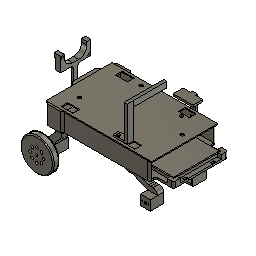
NatBot_V1 (Autodesk Fusion 360 design; units mm, degrees)
Autodesk Fusion 360 part; units mm, degrees
note: some values were not read from the file. Set by a fixed rule: which face or edge a step refers to.
(part 1 of 5)
sketch "MiniBot_v1" plane through (0, 0, 0) normal (0, 1, 0) x (1, 0, 0)
  line L0 (130.81, 3.81) -> (114.3, 3.81)
  circle A0 centre (147.6502, 58.6486) radius 2.54
  line L1 (114.3, 3.81) -> (114.3, 13.97)
  line L2 (130.81, 13.97) -> (130.81, 3.81)
  line L3 (114.3, 13.97) -> (130.81, 13.97)
  circle A1 centre (21.2344, 29.4894) radius 2.54
  line L4 (0, 0) -> (160, 0)
  line L5 (114.3, 86.36) -> (114.3, 96.52)
  line L6 (19.05, 96.52) -> (36.83, 96.52)
  line L7 (160, 0) -> (160, 100)
  line L8 (114.3, 96.52) -> (130.81, 96.52)
  line L9 (36.83, 96.52) -> (36.83, 86.36)
  circle A2 centre (102.5398, 7.1374) radius 2.54
  line L10 (36.83, 13.97) -> (36.83, 3.81)
  line L11 (19.05, 13.97) -> (36.83, 13.97)
  line L12 (19.05, 86.36) -> (19.05, 96.52)
  line L13 (36.83, 3.81) -> (19.05, 3.81)
  line L14 (130.81, 86.36) -> (114.3, 86.36)
  line L15 (19.05, 3.81) -> (19.05, 13.97)
  line L16 (130.81, 96.52) -> (130.81, 86.36)
  circle A3 centre (122.9106, 82.4992) radius 2.54
  line L17 (160, 100) -> (0, 100)
  line L18 (36.83, 86.36) -> (19.05, 86.36)
  circle A4 centre (52.2224, 92.0496) radius 2.54
  line L19 (0, 100) -> (0, 0)
extrude "Extrude1" add sketch "MiniBot_v1" along normal blind 1.57 makes body 1
sketch "Sketch1" plane through (0, 0, 0) normal (0, -1, 0) x (1, 0, 0) in component "battery"
  line L0 (19.05, -3.81) -> (36.83, -3.81)
  line L1 (36.83, -3.81) -> (36.83, -13.97)
  line L2 (36.83, -13.97) -> (19.05, -13.97)
  line L3 (19.05, -13.97) -> (19.05, -3.81)
  circle A0 centre (122.9106, -82.4992) radius 2.54
  circle A1 centre (52.2224, -92.0496) radius 2.54
  line L4 (130.81, -96.52) -> (114.3, -96.52)
  line L5 (114.3, -96.52) -> (114.3, -86.36)
  line L6 (114.3, -86.36) -> (130.81, -86.36)
  line L7 (130.81, -86.36) -> (130.81, -96.52)
  line L8 (36.83, -86.36) -> (36.83, -96.52)
  line L9 (36.83, -96.52) -> (19.05, -96.52)
  line L10 (19.05, -96.52) -> (19.05, -86.36)
  line L11 (19.05, -86.36) -> (36.83, -86.36)
  circle A2 centre (102.5398, -7.1374) radius 2.54
  circle A3 centre (21.2344, -29.4894) radius 2.54
  circle A4 centre (147.6502, -58.6486) radius 2.54
  line L12 (114.3, -13.97) -> (114.3, -3.81)
  line L13 (114.3, -3.81) -> (130.81, -3.81)
  line L14 (130.81, -3.81) -> (130.81, -13.97)
  line L15 (130.81, -13.97) -> (114.3, -13.97)
  line L16 (0, 0) -> (0, -100)
  line L17 (0, -100) -> (160, -100)
  line L18 (160, -100) -> (160, 0)
  line L19 (160, 0) -> (0, 0)
  line L20 (174, 0) -> (224.77, 0)
  line L21 (224.77, 0) -> (224.77, -71)
  line L22 (224.77, -71) -> (174, -71)
  line L23 (174, -71) -> (174, 0)
  dimension "d3" = 50.77
  dimension "d4" = 71
  constraint horizontal L20
  constraint vertical L21
  constraint horizontal L22
  constraint vertical L23
  measures "d3" distance of L20.start L20.end
  measures "d4" distance of L20.end L21.end
extrude "Extrude1'" add sketch "Sketch1" along normal blind 6 separate body contours L20 L21 L22 L23 makes body 2 in component "battery"
sketch "Sketch1 (2)" plane through (0, 0, 0) normal (0, -1, 0) x (1, 0, 0) in component "Arduino"
  line L0 (19.05, -3.81) -> (36.83, -3.81)
  line L1 (36.83, -3.81) -> (36.83, -13.97)
  line L2 (36.83, -13.97) -> (19.05, -13.97)
  line L3 (19.05, -13.97) -> (19.05, -3.81)
  circle A0 centre (122.9106, -82.4992) radius 2.54
  circle A1 centre (52.2224, -92.0496) radius 2.54
  line L4 (130.81, -96.52) -> (114.3, -96.52)
  line L5 (114.3, -96.52) -> (114.3, -86.36)
  line L6 (114.3, -86.36) -> (130.81, -86.36)
  line L7 (130.81, -86.36) -> (130.81, -96.52)
  line L8 (36.83, -86.36) -> (36.83, -96.52)
  line L9 (36.83, -96.52) -> (19.05, -96.52)
  line L10 (19.05, -96.52) -> (19.05, -86.36)
  line L11 (19.05, -86.36) -> (36.83, -86.36)
  circle A2 centre (102.5398, -7.1374) radius 2.54
  circle A3 centre (21.2344, -29.4894) radius 2.54
  circle A4 centre (147.6502, -58.6486) radius 2.54
  line L12 (114.3, -13.97) -> (114.3, -3.81)
  line L13 (114.3, -3.81) -> (130.81, -3.81)
  line L14 (130.81, -3.81) -> (130.81, -13.97)
  line L15 (130.81, -13.97) -> (114.3, -13.97)
  line L16 (0, 0) -> (0, -100)
  line L17 (0, -100) -> (160, -100)
  line L18 (160, -100) -> (160, 0)
  line L19 (160, 0) -> (0, 0)
  line L20 (92.1, -65.68) -> (38.1, -65.68)
  line L21 (38.1, -65.68) -> (38.1, -27.68)
  line L22 (38.1, -27.68) -> (92.1, -27.68)
  line L23 (92.1, -27.68) -> (92.1, -65.68)
  line L24 (92.1, -65.68) -> (38.1, -27.68) construction
  line L25 (38.1, -65.68) -> (92.1, -27.68) construction
  point P0 (65.1, -46.68)
  dimension "d7" = 54
  dimension "d8" = 38
  dimension "d9" = 27.68
  dimension "d10" = 38.1
  constraint horizontal L20
  constraint perpendicular L20 L21
  constraint parallel L20 L22
  constraint parallel L21 L23
  constraint coincident L24 P0
  constraint coincident L25 P0
  measures "d7" distance of L21.end L22.end
  measures "d8" distance of L20.end L21.end
  measures "d9" distance of L19 L22
  measures "d10" distance of L16 L21
extrude "Extrude1''" add sketch "Sketch1 (2)" along normal blind 11.3 separate body contours L20 L21 L22 L23 makes body 3 in component "Arduino"
fillet "Fillet1" radius 1 12 edges at (224.77, 0, -35.5) (224.77, -6, -35.5) (224.77, -3, 0) (199.385, 0, 0) (199.385, -6, 0) (199.385, 0, -71) (224.77, -3, -71) (199.385, -6, -71) (174, -3, -71) (174, -6, -35.5) (174, 0, -35.5) (174, -3, 0) on bodies 2 in component "battery"
sketch "Sketch2" plane through (0, -11.3, 0) normal (0, -1, 0) x (1, 0, 0) in component "Arduino"
  line L0 (92.1, -27.68) -> (38.1, -27.68)
  line L1 (38.1, -27.68) -> (38.1, -65.68)
  line L2 (38.1, -65.68) -> (92.1, -65.68)
  line L3 (92.1, -65.68) -> (92.1, -27.68)
  circle A0 centre (90.3, -50.39) radius 1.5
  circle A1 centre (50.7, -57.2) radius 1.5
  dimension "d14" = 3
  dimension "d15" = 3
  dimension "d16" = 8.48
  dimension "d17" = 12.6
  dimension "d18" = 1.8
  dimension "d22" = 22.71
  measures "d14" diameter of A0
  measures "d15" diameter of A1
  measures "d16" distance of L2 A1.centre
  measures "d17" distance of L1 A1.centre
  measures "d18" distance of L3 A0.centre
  measures "d22" distance of L0 A0.centre
extrude "Extrude2" cut sketch "Sketch2" against normal blind 2 contours A0 | A1 bodies 3 in component "Arduino"
sketch "Sketch2 (2)" plane through (0, 0, 0) normal (0, -1, 0) x (1, 0, 0) in component "Chassis"
  line L0 (19.05, -3.81) -> (36.83, -3.81)
  line L1 (36.83, -3.81) -> (36.83, -13.97)
  line L2 (36.83, -13.97) -> (19.05, -13.97)
  line L3 (19.05, -13.97) -> (19.05, -3.81)
  circle A0 centre (122.9106, -82.4992) radius 2.54
  circle A1 centre (52.2224, -92.0496) radius 2.54
  line L4 (130.81, -96.52) -> (114.3, -96.52)
  line L5 (114.3, -96.52) -> (114.3, -86.36)
  line L6 (114.3, -86.36) -> (130.81, -86.36)
  line L7 (130.81, -86.36) -> (130.81, -96.52)
  line L8 (36.83, -86.36) -> (36.83, -96.52)
  line L9 (36.83, -96.52) -> (19.05, -96.52)
  line L10 (19.05, -96.52) -> (19.05, -86.36)
  line L11 (19.05, -86.36) -> (36.83, -86.36)
  circle A2 centre (102.5398, -7.1374) radius 2.54
  circle A3 centre (21.2344, -29.4894) radius 2.54
  circle A4 centre (147.6502, -58.6486) radius 2.54
  line L12 (114.3, -13.97) -> (114.3, -3.81)
  line L13 (114.3, -3.81) -> (130.81, -3.81)
  line L14 (130.81, -3.81) -> (130.81, -13.97)
  line L15 (130.81, -13.97) -> (114.3, -13.97)
  line L16 (0, 0) -> (0, -100)
  line L17 (0, -100) -> (160, -100)
  line L18 (160, -100) -> (160, 0)
  line L19 (160, 0) -> (0, 0)
sketch "Sketch3" plane through (0, 0, 0) normal (0, -1, 0) x (1, 0, 0) in component "Chassis"
  circle A0 centre (21.2344, -29.4894) radius 2.54 construction
  circle A1 centre (102.5398, -7.1374) radius 2.54
  circle A2 centre (147.6502, -58.6486) radius 2.54
  circle A3 centre (122.9106, -82.4992) radius 2.54
  circle A4 centre (52.2224, -92.0496) radius 2.54
  circle A5 centre (21.2344, -29.4894) radius 5
  circle A6 centre (102.5398, -7.1374) radius 5
  circle A7 centre (147.6502, -58.6486) radius 5
  circle A8 centre (122.9106, -82.4992) radius 5
  circle A9 centre (52.2224, -92.0496) radius 5
  dimension "d23" = 10
  dimension "d24" = 10
  dimension "d25" = 10
  dimension "d26" = 10
  dimension "d27" = 10
  constraint concentric A0 A5
  constraint concentric A1 A6
  constraint concentric A2 A7
  constraint concentric A3 A8
  constraint concentric A4 A9
  measures "d23" diameter of A5
  measures "d24" diameter of A6
  measures "d25" diameter of A7
  measures "d26" diameter of A8
  measures "d27" diameter of A9
extrude "Extrude1'''" add sketch "Sketch3" along normal blind 23.65 separate body contours A1 | A3 | A4 | A5 | A6 | A8 | A9 makes body 4 at (26.2096, -7.8833, -29.9872) makes body 5 at (57.1976, -7.8833, -92.5474) makes body 6 at (107.515, -7.8833, -7.6352) makes body 7 at (127.8858, -7.8833, -82.997) in component "Chassis"
sketch "Sketch4" plane through (0, 0, 0) normal (0, 1, 0) x (1, 0, 0) in component "Chassis"
  line L0 (0, 0) -> (160, 0)
  line L1 (0, 100) -> (0, 0)
  line L2 (160, 100) -> (0, 100)
  line L3 (160, 0) -> (160, 100)
  line L4 (157, 97) -> (3, 97)
  line L5 (3, 97) -> (3, 3)
  line L6 (3, 3) -> (157, 3)
  line L7 (157, 3) -> (157, 97)
  line L8 (157, 3) -> (157, 0)
  line L9 (157, 97) -> (157, 100)
  dimension "d32" = -3
  constraint coincident L0 L8.end
  constraint perpendicular L0 L8
  constraint coincident L2 L9.end
  constraint perpendicular L2 L9
extrude "Extrude2'" add sketch "Sketch4" against normal blind 23.65 contours L0 L1 L2 L4 L5 L6 L8 L9 bodies 5 6 in component "Chassis"
sketch "Sketch5" plane through (0, -11.3, 0) normal (0, -1, 0) x (1, 0, 0) in component "Chassis"
  circle A0 centre (50.7, -57.2) radius 1.5
  circle A1 centre (90.3, -50.39) radius 1.5
  line L0 (92.1, -27.68) -> (38.1, -27.68)
  line L1 (38.1, -27.68) -> (38.1, -65.68)
  line L2 (38.1, -65.68) -> (92.1, -65.68)
  line L3 (92.1, -65.68) -> (92.1, -27.68)
  line L4 (65.1, -27.68) -> (65.1, -65.68) construction
  line L5 (38.1, -46.68) -> (92.1, -46.68) construction
  line L6 (80.1, -54.18) -> (50.1, -54.18)
  line L7 (50.1, -54.18) -> (50.1, -39.18)
  line L8 (50.1, -39.18) -> (80.1, -39.18)
  line L9 (80.1, -39.18) -> (80.1, -54.18)
  line L10 (80.1, -54.18) -> (50.1, -39.18) construction
  line L11 (50.1, -54.18) -> (80.1, -39.18) construction
  point P0 (65.1, -46.68)
  dimension "d35" = 30
  dimension "d36" = 15
  constraint midpoint L0 L4.start
  constraint midpoint L2 L4.end
  constraint midpoint L1 L5.start
  constraint midpoint L3 L5.end
  constraint horizontal L6
  constraint perpendicular L6 L7
  constraint parallel L6 L8
  constraint parallel L7 L9
  constraint coincident L10 P0
  constraint coincident L11 P0
  constraint midpoint L4 P0
  measures "d35" distance of L7.end L8.end
  measures "d36" distance of L6.end L7.end
extrude "Extrude3" add sketch "Sketch5" along normal blind 12.35 separate body contours L6 L7 L8 L9 makes body 8 in component "Chassis"
sketch "Sketch7" plane through (0, -23.65, 0) normal (0, -1, 0) x (1, 0, 0) in component "Chassis"
  line L0 (105.3473, -3) -> (157, -3)
  line L1 (157, -3) -> (157, 0)
  line L2 (157, 0) -> (0, 0)
  line L3 (0, 0) -> (0, -100)
  line L4 (0, -100) -> (157, -100)
  line L5 (157, -100) -> (157, -97)
  line L6 (157, -97) -> (52.9249, -97)
  arc A0 (52.9249, -97) -> (51.5199, -97) centre (52.2224, -92.0496) ccw
  line L7 (51.5199, -97) -> (3, -97)
  line L8 (3, -97) -> (3, -3)
  line L9 (3, -3) -> (99.7323, -3)
  arc A1 (99.7323, -3) -> (105.3473, -3) centre (102.5398, -7.1374) ccw
  line L10 (0, 0) -> (157, 0)
  line L11 (157, 0) -> (157, -100)
  line L12 (157, -100) -> (0, -100)
  line L13 (0, -100) -> (0, 0)
  constraint horizontal L10
  constraint vertical L11
  constraint horizontal L12
  constraint vertical L13
  constraint coincident L4.end L5.start
  constraint coincident L2.end L3.start
extrude "Extrude4" add sketch "Sketch7" along normal blind 3 bodies 4 5 7 8 in component "Chassis"
extrude "Extrude5" cut sketch "MiniBot_v1" against normal blind 26.65 contours L0 L1 L2 L3 | L5 L8 L14 L16 | L6 L9 L12 L18 | L10 L11 L13 L15 bodies 4 in component "Chassis"
sketch "Sketch8" plane through (0, 0, 0) normal (0, 1, 0) x (-1, 0, 0) in component "Chassis"
  line L0 (-99.7323, -3) -> (-3, -3)
  line L1 (-3, -3) -> (-3, -97)
  line L2 (-3, -97) -> (-51.5199, -97)
  arc A0 (-51.5199, -97) -> (-52.9249, -97) centre (-52.2224, -92.0496) ccw
  line L3 (-52.9249, -97) -> (-157, -97)
  line L4 (-157, -97) -> (-157, -100)
  line L5 (-157, -100) -> (0, -100)
  line L6 (0, -100) -> (0, 0)
  line L7 (0, 0) -> (-157, 0)
  line L8 (-157, 0) -> (-157, -3)
  line L9 (-157, -3) -> (-105.3473, -3)
  arc A1 (-105.3473, -3) -> (-99.7323, -3) centre (-102.5398, -7.1374) ccw
  circle A2 centre (-102.5398, -7.1374) radius 3.135
  circle A3 centre (-52.2224, -92.0496) radius 3.135
  dimension "d43" = 6.27
  dimension "d44" = 6.27
  constraint concentric A1 A2
  constraint concentric A0 A3
  measures "d43" diameter of A2
  measures "d44" diameter of A3
extrude "Extrude6" cut sketch "Sketch8" against normal blind 5.96 contours A2 | A3 bodies 4 in component "Chassis"
sketch "Sketch9" plane through (0, 0, 0) normal (0, 1, 0) x (-1, 0, 0) in component "Chassis"
  circle A0 centre (-21.2344, -29.4894) radius 5
  circle A1 centre (-21.2344, -29.4894) radius 3.135
  dimension "d47" = 6.27
  constraint concentric A0 A1
  measures "d47" diameter of A1
extrude "Extrude7" cut sketch "Sketch9" against normal blind 5.96 contours A1 bodies 4 in component "Chassis"
sketch "Sketch10" plane through (0, 0, 0) normal (0, 1, 0) x (-1, 0, 0) in component "Chassis"
  line L0 (-126.0877, -86.36) -> (-119.7335, -86.36)
  arc A0 (-119.7335, -86.36) -> (-126.0877, -86.36) centre (-122.9106, -82.4992) ccw
  circle A1 centre (-122.9106, -82.4992) radius 3.135
  dimension "d50" = 6.27
  constraint concentric A0 A1
  measures "d50" diameter of A1
extrude "Extrude8" cut sketch "Sketch10" against normal blind 5.96 contours A1 bodies 4 in component "Chassis"
sketch "Sketch11" plane through (157, 0, 0) normal (1, 0, 0) x (0, 0, -1) in component "Chassis"
  line L0 (0, 0) -> (0, -26.65)
  line L1 (0, -26.65) -> (100, -26.65)
  line L2 (100, -26.65) -> (100, 0)
  line L3 (100, 0) -> (97, 0)
  line L4 (97, 0) -> (97, -23.65)
  line L5 (97, -23.65) -> (3, -23.65)
  line L6 (3, -23.65) -> (3, 0)
  line L7 (3, 0) -> (0, 0)
  arc A0 (84.5, -23.65) -> (85.5, -22.65) centre (84.5, -22.65) ccw
  line L8 (85.5, -22.65) -> (85.5, -18.65)
  arc A1 (85.5, -18.65) -> (84.5, -17.65) centre (84.5, -18.65) ccw
  line L9 (85.5, -22.65) -> (85.5, -26.65) construction
  arc A2 (15.5, -17.65) -> (14.5, -18.65) centre (15.5, -18.65) ccw
  line L10 (14.5, -18.65) -> (14.5, -22.65)
  arc A3 (14.5, -22.65) -> (15.5, -23.65) centre (15.5, -22.65) ccw
  line L11 (14.5, -22.65) -> (14.5, -26.65) construction
  line L12 (14.5, -23.65) -> (9, -23.65)
  line L13 (85.5, -26.65) -> (91, -26.65)
  line L14 (9, -23.65) -> (91, -23.65)
  line L15 (91, -23.65) -> (91, -26.65)
  line L16 (91, -26.65) -> (9, -26.65)
  line L17 (9, -26.65) -> (9, -23.65)
  constraint coincident A0.end L8.start
  constraint coincident L1 L9.end
  constraint tangent A0 L9
  constraint coincident L10.end A3.start
  constraint coincident L1 L11.end
  constraint tangent A3 L11
  constraint coincident L11 L12.start
  constraint coincident L5 L12.start
  constraint coincident L5 L12.end
  constraint perpendicular L0 L12
  constraint coincident L1 L13.end
  constraint perpendicular L9 L13
  constraint horizontal L14
  constraint vertical L15
  constraint horizontal L16
  constraint vertical L17
extrude "Extrude9" add sketch "Sketch11" along normal blind 27.27 contours L1 L5 L12 L13 L14 L15 L16 L17 bodies 4 in component "Chassis"
sketch "Sketch12" plane through (0, -23.65, 0) normal (0, 1, 0) x (-1, 0, 0) in component "Chassis"
  line L0 (-130.81, -86.36) -> (-126.0877, -86.36)
  arc A0 (-119.7335, -86.36) -> (-126.0877, -86.36) centre (-122.9106, -82.4992) ccw
  line L1 (-119.7335, -86.36) -> (-114.3, -86.36)
  line L2 (-114.3, -86.36) -> (-114.3, -96.52)
  line L3 (-114.3, -96.52) -> (-130.81, -96.52)
  line L4 (-130.81, -96.52) -> (-130.81, -86.36)
  line L5 (-36.83, -13.97) -> (-36.83, -3.81)
  line L6 (-36.83, -3.81) -> (-19.05, -3.81)
  line L7 (-19.05, -3.81) -> (-19.05, -13.97)
  line L8 (-19.05, -13.97) -> (-36.83, -13.97)
  line L9 (-19.05, -96.52) -> (-36.83, -96.52)
  line L10 (-36.83, -96.52) -> (-36.83, -86.36)
  line L11 (-36.83, -86.36) -> (-19.05, -86.36)
  line L12 (-19.05, -86.36) -> (-19.05, -96.52)
  line L13 (-130.81, -3.81) -> (-114.3, -3.81)
  line L14 (-114.3, -3.81) -> (-114.3, -13.97)
  line L15 (-114.3, -13.97) -> (-130.81, -13.97)
  line L16 (-130.81, -13.97) -> (-130.81, -3.81)
  line L17 (-80.1, -54.18) -> (-80.1, -39.18)
  line L18 (-80.1, -39.18) -> (-50.1, -39.18)
  line L19 (-50.1, -39.18) -> (-50.1, -54.18)
  line L20 (-50.1, -54.18) -> (-80.1, -54.18)
  line L21 (-105.3473, -3) -> (-157, -3)
  line L22 (-157, -3) -> (-157, -9)
  line L23 (-157, -9) -> (-184.27, -9)
  line L24 (-184.27, -9) -> (-184.27, -91)
  line L25 (-184.27, -91) -> (-157, -91)
  line L26 (-157, -91) -> (-157, -97)
  line L27 (-157, -97) -> (-52.9249, -97)
  arc A1 (-51.5199, -97) -> (-52.9249, -97) centre (-52.2224, -92.0496) ccw
  line L28 (-51.5199, -97) -> (-3, -97)
  line L29 (-3, -97) -> (-3, -3)
  line L30 (-3, -3) -> (-99.7323, -3)
  arc A2 (-105.3473, -3) -> (-99.7323, -3) centre (-102.5398, -7.1374) ccw
  circle A3 centre (-21.2344, -29.4894) radius 5
  line L31 (-184.27, -9) -> (-174.27, -9)
  line L32 (-184.27, -9) -> (-184.27, -19)
  line L33 (-174.27, -9) -> (-174.27, -14.4)
  line L34 (-184.27, -19) -> (-178.87, -19)
  line L35 (-178.87, -19) -> (-178.8806, -9) construction
  line L36 (-174.27, -14.4) -> (-178.8749, -14.4049)
  line L37 (-178.87, -19) -> (-178.8749, -14.4049)
  line L38 (-184.27, -50) -> (-180, -50) construction
  line L39 (-184.27, -91) -> (-174.27, -91)
  line L40 (-184.27, -91) -> (-184.27, -81)
  line L41 (-174.27, -91) -> (-174.27, -85.6)
  line L42 (-174.27, -85.6) -> (-178.8749, -85.5951)
  line L43 (-178.87, -81) -> (-178.8749, -85.5951)
  line L44 (-184.27, -81) -> (-178.87, -81)
  line L45 (-127.9, -50) -> (-127.9, -46) construction
  line L46 (-127.9, -50) -> (-127.9, -54) construction
  line L47 (-128, -84.5) -> (-128, -15.5)
  line L48 (-127.9, -54) -> (-125.4, -54) construction
  line L49 (-127.9, -46) -> (-125.4, -46)
  line L50 (-125.4, -46) -> (-125.4, -54)
  line L51 (-125.4, -54) -> (-127.9, -54)
  line L52 (-127.9, -54) -> (-127.9, -46)
  dimension "d55" = 10
  dimension "d56" = 10
  dimension "d57" = 5.4
  dimension "d58" = 5.4
  dimension "d59" = 4.5951
  dimension "d60" = 0.1
  dimension "d61" = 2.5
  constraint coincident L23.end L24.start
  constraint perpendicular L24 L31
  constraint perpendicular L23 L32
  constraint perpendicular L23 L33
  constraint perpendicular L24 L34
  constraint coincident L23 L35.end
  constraint coincident L35 L36.end
  constraint perpendicular L35 L36
  constraint midpoint L24 L38.start
  constraint perpendicular L24 L38
  constraint symmetric L23.end L38 L24.end
  constraint symmetric L31.end L38 L39.end
  constraint symmetric L32.end L38 L40.end
  constraint symmetric L33.end L38 L41.end
  constraint symmetric L34.end L38 L43.start
  constraint symmetric L36.end L38 L42.end
  constraint parallel L17 L45
  constraint parallel L45 L46
  constraint perpendicular L46 L48
  constraint horizontal L49
  constraint vertical L50
  constraint horizontal L51
  constraint vertical L52
  measures "d55" distance of L23.end L31.end
  measures "d56" distance of L23.end L32.end
  measures "d57" distance of L31.end L33.end
  measures "d58" distance of L32.end L34.end
  measures "d59" vertical distance of L34.end L36.end
  measures "d60" distance of L45 L47
  measures "d61" distance of L46.end L48.end
extrude "Extrude10" add sketch "Sketch12" along normal blind 6 contours L23 L24 L31 L32 L33 L34 L36 L37 | L24 L25 L39 L40 L41 L42 L43 L44 | L49 L50 L51 L52 bodies 4 in component "Chassis"
fillet "Fillet1'" radius 3 4 edges at (184.27, -22.15, -9) (157, -25.15, -9) (157, -25.15, -91) (184.27, -22.15, -91) on bodies 4 in component "Chassis"
fillet "Fillet2" radius 3 2 edges at (0, -13.325, 0) (0, -13.325, -100) on bodies 4 in component "Chassis"
fillet "Fillet3" radius 3 2 edges at (157, -13.325, -100) (157, -13.325, 0) on bodies 4 in component "Chassis"
extrude "Extrude11" cut 1 faces at (60.1, -11.3, -49.18) along direction (0, -1, 0) blind 1 on bodies 4 bodies 4 in component "Chassis"
fillet "Fillet4" radius 3 4 edges at (80.1, -17.975, -39.18) (50.1, -17.975, -39.18) (80.1, -17.975, -54.18) (50.1, -17.975, -54.18) on bodies 4 in component "Chassis"
fillet "Fillet5" radius 3 2 edges at (3, -11.825, -97) (3, -11.825, -3) on bodies 4 in component "Chassis"
sketch "Sketch13" plane through (0, -23.65, 0) normal (0, 1, 0) x (-1, 0, 0) in component "Chassis"
  arc A0 (-3, -6) -> (-6, -3) centre (-6, -6) ccw
  line L0 (-6, -3) -> (-99.7323, -3)
  arc A1 (-105.3473, -3) -> (-99.7323, -3) centre (-102.5398, -7.1374) ccw
  line L1 (-105.3473, -3) -> (-157, -3)
  line L2 (-157, -3) -> (-157, -6)
  arc A2 (-160, -9) -> (-157, -6) centre (-160, -6) ccw
  line L3 (-160, -9) -> (-174.27, -9)
  line L4 (-174.27, -9) -> (-174.27, -14.4)
  line L5 (-174.27, -14.4) -> (-178.8749, -14.4049)
  line L6 (-178.8749, -14.4049) -> (-178.87, -19)
  line L7 (-178.87, -19) -> (-184.27, -19)
  line L8 (-184.27, -19) -> (-184.27, -81)
  line L9 (-184.27, -81) -> (-178.87, -81)
  line L10 (-178.87, -81) -> (-178.8749, -85.5951)
  line L11 (-178.8749, -85.5951) -> (-174.27, -85.6)
  line L12 (-174.27, -85.6) -> (-174.27, -91)
  line L13 (-174.27, -91) -> (-160, -91)
  arc A3 (-157, -94) -> (-160, -91) centre (-160, -94) ccw
  line L14 (-157, -94) -> (-157, -97)
  line L15 (-157, -97) -> (-52.9249, -97)
  arc A4 (-51.5199, -97) -> (-52.9249, -97) centre (-52.2224, -92.0496) ccw
  line L16 (-51.5199, -97) -> (-6, -97)
  arc A5 (-6, -97) -> (-3, -94) centre (-6, -94) ccw
  line L17 (-3, -94) -> (-3, -6)
  line L18 (-127.9, -54) -> (-127.9, -46)
  line L19 (-127.9, -46) -> (-125.4, -46)
  line L20 (-125.4, -46) -> (-125.4, -54)
  line L21 (-125.4, -54) -> (-127.9, -54)
  line L22 (-130.81, -86.36) -> (-126.0877, -86.36)
  arc A6 (-119.7335, -86.36) -> (-126.0877, -86.36) centre (-122.9106, -82.4992) ccw
  line L23 (-119.7335, -86.36) -> (-114.3, -86.36)
  line L24 (-114.3, -86.36) -> (-114.3, -96.52)
  line L25 (-114.3, -96.52) -> (-130.81, -96.52)
  line L26 (-130.81, -96.52) -> (-130.81, -86.36)
  line L27 (-36.83, -13.97) -> (-36.83, -3.81)
  line L28 (-36.83, -3.81) -> (-19.05, -3.81)
  line L29 (-19.05, -3.81) -> (-19.05, -13.97)
  line L30 (-19.05, -13.97) -> (-36.83, -13.97)
  line L31 (-19.05, -96.52) -> (-36.83, -96.52)
  line L32 (-36.83, -96.52) -> (-36.83, -86.36)
  line L33 (-36.83, -86.36) -> (-19.05, -86.36)
  line L34 (-19.05, -86.36) -> (-19.05, -96.52)
  line L35 (-130.81, -3.81) -> (-114.3, -3.81)
  line L36 (-114.3, -3.81) -> (-114.3, -13.97)
  line L37 (-114.3, -13.97) -> (-130.81, -13.97)
  line L38 (-130.81, -13.97) -> (-130.81, -3.81)
  line L39 (-80.1, -51.18) -> (-80.1, -42.18)
  arc A7 (-77.1, -39.18) -> (-80.1, -42.18) centre (-77.1, -42.18) ccw
  line L40 (-77.1, -39.18) -> (-53.1, -39.18)
  arc A8 (-50.1, -42.18) -> (-53.1, -39.18) centre (-53.1, -42.18) ccw
  line L41 (-50.1, -42.18) -> (-50.1, -51.18)
  arc A9 (-53.1, -54.18) -> (-50.1, -51.18) centre (-53.1, -51.18) ccw
  line L42 (-53.1, -54.18) -> (-77.1, -54.18)
  arc A10 (-80.1, -51.18) -> (-77.1, -54.18) centre (-77.1, -51.18) ccw
  circle A11 centre (-21.2344, -29.4894) radius 5
  line L43 (-184.27, -19) -> (-184.27, -29) construction
  line L44 (-184.27, -81) -> (-184.27, -71) construction
  line L45 (-184.27, -29) -> (-182, -29) construction
  line L46 (-184.27, -71) -> (-182, -71) construction
  line L47 (-183.5, -31.5) -> (-180.5, -31.5)
  line L48 (-180.5, -31.5) -> (-180.5, -26.5)
  line L49 (-180.5, -26.5) -> (-183.5, -26.5)
  line L50 (-183.5, -26.5) -> (-183.5, -31.5)
  line L51 (-183.5, -31.5) -> (-180.5, -26.5) construction
  line L52 (-180.5, -31.5) -> (-183.5, -26.5) construction
  line L53 (-183.5, -73.5) -> (-180.5, -73.5)
  line L54 (-180.5, -73.5) -> (-180.5, -68.5)
  line L55 (-180.5, -68.5) -> (-183.5, -68.5)
  line L56 (-183.5, -68.5) -> (-183.5, -73.5)
  line L57 (-183.5, -73.5) -> (-180.5, -68.5) construction
  line L58 (-180.5, -73.5) -> (-183.5, -68.5) construction
  line L59 (-182, -29) -> (-126, -29) construction
  line L60 (-182, -71) -> (-126, -71) construction
  line L61 (-127.5, -31.5) -> (-124.5, -31.5)
  line L62 (-124.5, -31.5) -> (-124.5, -26.5)
  line L63 (-124.5, -26.5) -> (-127.5, -26.5)
  line L64 (-127.5, -26.5) -> (-127.5, -31.5)
  line L65 (-127.5, -31.5) -> (-124.5, -26.5) construction
  line L66 (-124.5, -31.5) -> (-127.5, -26.5) construction
  line L67 (-127.5, -73.5) -> (-124.5, -73.5)
  line L68 (-124.5, -73.5) -> (-124.5, -68.5)
  line L69 (-124.5, -68.5) -> (-127.5, -68.5)
  line L70 (-127.5, -68.5) -> (-127.5, -73.5)
  line L71 (-127.5, -73.5) -> (-124.5, -68.5) construction
  line L72 (-124.5, -73.5) -> (-127.5, -68.5) construction
  point P0 (-182, -29)
  point P1 (-182, -71)
  point P2 (-126, -29)
  point P3 (-126, -71)
  dimension "d71" = 10
  dimension "d72" = 10
  dimension "d73" = 3
  dimension "d74" = 5
  dimension "d75" = 3
  dimension "d76" = 5
  dimension "d77" = 3
  dimension "d78" = 5
  dimension "d79" = 3
  dimension "d80" = 5
  constraint coincident L7.end L8.start
  constraint perpendicular L7 L43
  constraint coincident L8.end L9.start
  constraint perpendicular L9 L44
  constraint perpendicular L8 L45
  constraint perpendicular L44 L46
  constraint horizontal L47
  constraint perpendicular L47 L48
  constraint parallel L47 L49
  constraint parallel L48 L50
  constraint coincident L51 P0
  constraint coincident L52 P0
  constraint coincident P0 L45.end
  constraint horizontal L53
  constraint perpendicular L53 L54
  constraint parallel L53 L55
  constraint parallel L54 L56
  constraint coincident L57 P1
  constraint coincident L58 P1
  constraint coincident P1 L46.end
  constraint parallel L49 L59
  constraint parallel L21 L60
  constraint horizontal L61
  constraint perpendicular L61 L62
  constraint parallel L61 L63
  constraint parallel L62 L64
  constraint coincident L65 P2
  constraint coincident L66 P2
  constraint coincident P2 L59.end
  constraint horizontal L67
  constraint perpendicular L67 L68
  constraint parallel L67 L69
  constraint parallel L68 L70
  constraint coincident L71 P3
  constraint coincident L72 P3
  constraint coincident P3 L60.end
  measures "d71" distance of L7.end L43.end
  measures "d72" distance of L8.end L44.end
  measures "d73" distance of L48.end L49.end
  measures "d74" distance of L47.end L48.end
  measures "d75" distance of L54.end L55.end
  measures "d76" distance of L53.end L54.end
  measures "d77" distance of L62.end L63.end
  measures "d78" distance of L61.end L62.end
  measures "d79" distance of L68.end L69.end
  measures "d80" distance of L67.end L68.end
extrude "Extrude12" cut sketch "Sketch13" against normal blind 3 contours L47 L48 L49 L50 | L53 L54 L55 L56 | L61 L62 L63 L64 | L67 L68 L69 L70 bodies 4 in component "Chassis"
sketch "Sketch14" plane through (0, 0, 0) normal (0, 1, 0) x (-1, 0, 0) in component "Chassis"
  circle A0 centre (-52.2224, -92.0496) radius 3.135
  circle A1 centre (-102.5398, -7.1374) radius 3.135
  arc A2 (-154, 0) -> (-157, -3) centre (-154, -3) ccw
  line L0 (-157, -3) -> (-105.3473, -3)
  arc A3 (-105.3473, -3) -> (-99.7323, -3) centre (-102.5398, -7.1374) ccw
  line L1 (-99.7323, -3) -> (-6, -3)
  arc A4 (-3, -6) -> (-6, -3) centre (-6, -6) ccw
  line L2 (-3, -6) -> (-3, -94)
  arc A5 (-6, -97) -> (-3, -94) centre (-6, -94) ccw
  line L3 (-6, -97) -> (-51.5199, -97)
  arc A6 (-51.5199, -97) -> (-52.9249, -97) centre (-52.2224, -92.0496) ccw
  line L4 (-52.9249, -97) -> (-157, -97)
  arc A7 (-157, -97) -> (-154, -100) centre (-154, -97) ccw
  line L5 (-154, -100) -> (-3, -100)
  arc A8 (-3, -100) -> (0, -97) centre (-3, -97) ccw
  line L6 (0, -97) -> (0, -3)
  arc A9 (0, -3) -> (-3, 0) centre (-3, -3) ccw
  line L7 (-3, 0) -> (-154, 0)
  line L8 (-3, -94) -> (0, -94)
  line L9 (0, -94) -> (0, -6)
  line L10 (0, -6) -> (-3, -6)
  line L11 (-3, -6) -> (-3, -94)
  constraint horizontal L8
  constraint vertical L9
  constraint horizontal L10
  constraint vertical L11
  constraint coincident L6 L9.end
  constraint coincident L2.end A5.end
extrude "Extrude13" cut sketch "Sketch14" against normal blind 2 contours L2 L6 L8 L9 L10 L11 bodies 4 in component "Chassis"
fillet "Fillet6" radius 2 2 edges at (1.5, -2, -94) (1.5, -2, -6) on bodies 4 in component "Chassis"
sketch "Sketch15" plane through (0, 0, -100) normal (0, 0, -1) x (-1, 0, 0) in component "Chassis"
  line L0 (-154, 0) -> (-154, -26.65)
  line L1 (-154, -26.65) -> (-3, -26.65)
  line L2 (-3, -26.65) -> (-3, 0)
  line L3 (-3, 0) -> (-154, 0)
  line L4 (-114.3178, 0) -> (-130.8159, 0) construction
  line L5 (-122.5668, 0) -> (-122.5668, -26.65) construction
  circle A0 centre (-122.5668, -5.65) radius 1.25
  circle A1 centre (-122.5668, -10.65) radius 1.25
  dimension "d86" = 2.5
  dimension "d87" = 2.5
  dimension "d88" = 5
  dimension "d89" = 16
  constraint coincident L3 L4.start
  constraint coincident L3 L4.end
  constraint parallel L3 L4
  constraint midpoint L4 L5.start
  constraint coincident L1 L5.end
  constraint perpendicular L1 L5
  constraint coincident L5 A0.centre
  constraint coincident L5 A1.centre
  measures "d86" diameter of A0
  measures "d87" diameter of A1
  measures "d88" distance of A0.centre A1.centre
  measures "d89" distance of L1 A1.centre
extrude "Extrude14" cut sketch "Sketch15" against normal blind 3 contours A0 | A1 bodies 4 in component "Chassis"
sketch "Sketch1 (3)" plane through (0, 0, -100) normal (0, 0, -1) x (-1, 0, 0) in component "GPS_Mount"
  circle A0 centre (-122.5668, -10.65) radius 1.25
  circle A1 centre (-122.5668, -5.65) radius 1.25
  line L0 (-154, 0) -> (-154, -26.65)
  line L1 (-154, -26.65) -> (-3, -26.65)
  line L2 (-3, -26.65) -> (-3, 0)
  line L3 (-3, 0) -> (-154, 0) construction
  line L4 (-122.5668, -5.65) -> (-122.5668, -10.65) construction
  line L5 (-122.5668, -8.15) -> (-125, -8.15) construction
  line L6 (-119, -13) -> (-126.1337, -13)
  circle A2 centre (-122.5668, -5.65) radius 1.375
  circle A3 centre (-122.5668, -10.65) radius 1.375
  line L7 (-126.1337, -13) -> (-126.1337, 22)
  line L8 (-126.1337, 22) -> (-119, 22)
  line L9 (-119, 22) -> (-119, -13)
  point P0 (-122.5668, -8.15)
  dimension "d92" = 2.75
  dimension "d93" = 2.75
  dimension "d101" = 35
  constraint coincident A1.centre L4.start
  constraint coincident A0.centre L4.end
  constraint midpoint L4 P0
  constraint perpendicular L4 L5
  constraint horizontal L6
  constraint coincident P0 L5.start
  constraint perpendicular L3 L7
  constraint perpendicular L7 L8
  constraint perpendicular L6 L9
  measures "d92" diameter of A2
  measures "d93" diameter of A3
  measures "d101" distance of L6.end L7.end
extrude "Extrude1''''" add sketch "Sketch1 (3)" along normal blind 3 separate body contours L6 L7 L8 L9 makes body 9 in component "GPS_Mount"
sketch "Sketch2 (3)" plane through (0, 0, -100) normal (0, 0, 1) x (1, 0, 0) in component "GPS_Mount"
  circle A0 centre (122.5668, -10.65) radius 1.375
  circle A1 centre (122.5668, -5.65) radius 1.375
  line L0 (126.1337, 22) -> (119, 22)
  line L1 (119, 22) -> (119, -13) construction
  line L2 (119, -13) -> (126.1337, -13)
  line L3 (126.1337, -13) -> (126.1337, 22) construction
  line L4 (126.1337, 19) -> (119, 19) construction
  line L5 (122.5668, 19) -> (107.5668, 19)
  line L6 (107.5668, 19) -> (107.5668, 22)
  line L7 (107.5668, 22) -> (122.5668, 22)
  line L8 (122.5668, 22) -> (122.5668, 19) construction
  line L9 (122.5668, 22) -> (137.5668, 22)
  line L10 (137.5668, 22) -> (137.5668, 19)
  line L11 (137.5668, 19) -> (122.5668, 19)
  line L12 (122.5668, 19) -> (122.5668, 22) construction
  dimension "d96" = 3
  dimension "d97" = 15
  dimension "d98" = 15
  constraint coincident L3 L4.start
  constraint coincident L1 L4.end
  constraint perpendicular L1 L4
  constraint horizontal L5
  constraint vertical L6
  constraint horizontal L7
  constraint vertical L8
  constraint midpoint L4 L5.start
  constraint horizontal L9
  constraint vertical L10
  constraint horizontal L11
  constraint vertical L12
  measures "d96" distance of L0 L4
  measures "d97" distance of L5.start L5.end
  measures "d98" distance of L7.end L9.end
extrude "Extrude2''" add sketch "Sketch2 (3)" along normal blind 15 contours L0 L5 L6 L7 L9 L10 L11 bodies 9 in component "GPS_Mount"
sketch "Sketch1 (4)" plane through (0, 0, 0) normal (-1, 0, 0) x (0, 0, 1) in component "Ultrasonic_Sensor_Mount"
  line L0 (-94, 0) -> (-97, 0)
  line L1 (-97, 0) -> (-97, -26.65)
  line L2 (-97, -26.65) -> (-3, -26.65)
  line L3 (-3, -26.65) -> (-3, 0)
  line L4 (-3, 0) -> (-6, 0)
  arc A0 (-8, -2) -> (-6, 0) centre (-8, 0) ccw
  line L5 (-8, -2) -> (-92, -2)
  arc A1 (-94, 0) -> (-92, -2) centre (-92, 0) ccw
  line L6 (-50, -2) -> (-50, -31) construction
  constraint midpoint L5 L6.start
  constraint perpendicular L2 L6
sketch "Sketch16" plane through (0, 0, 0) normal (-1, 0, 0) x (0, 0, 1) in component "Chassis"
  circle A0 centre (-50, -6.65) radius 1.375
  circle A1 centre (-50, -11.65) radius 1.375
  line L0 (-97, -26.65) -> (-3, -26.65)
  dimension "d102" = 2.75
  dimension "d103" = 2.75
  dimension "d104" = 5
  dimension "d105" = 15
  measures "d102" diameter of A0
  measures "d103" diameter of A1
  measures "d104" distance of A0.centre A1.centre
  measures "d105" distance of A1.centre L0
extrude "Extrude15" cut sketch "Sketch16" against normal blind 3 bodies 4 in component "Chassis"
sketch "Sketch2 (4)" plane through (0, 0, 0) normal (-1, 0, 0) x (0, 0, 1) in component "Ultrasonic_Sensor_Mount"
  circle A0 centre (-50, -6.65) radius 1.375
  circle A1 centre (-50, -11.65) radius 1.375
  circle A2 centre (-50, -6.65) radius 1.375
  circle A3 centre (-50, -11.65) radius 1.375
  line L0 (-53, -14) -> (-47, -14)
  line L1 (-53, -14) -> (-53, 22)
  line L2 (-53, 22) -> (-47, 22)
  line L3 (-47, 22) -> (-47, -14)
  point P0 (-50, -9.15)
  constraint concentric A0 A2
  constraint concentric A1 A3
  constraint horizontal L0
  constraint perpendicular L0 L1
  constraint perpendicular L1 L2
  constraint perpendicular L0 L3
extrude "Extrude1'''''" add sketch "Sketch2 (4)" along normal blind 3 separate body makes body 10 in component "Ultrasonic_Sensor_Mount"
sketch "Sketch3 (2)" plane through (-3, 0, 0) normal (-1, 0, 0) x (0, 0, 1) in component "Ultrasonic_Sensor_Mount"
  circle A0 centre (-50, -6.65) radius 1.375
  circle A1 centre (-50, -11.65) radius 1.375
  line L0 (-53, -14) -> (-47, -14)
  line L1 (-47, -14) -> (-47, 22)
  line L2 (-47, 22) -> (-53, 22)
  line L3 (-53, 22) -> (-53, -14)
  line L4 (-50, 22) -> (-27.15, 22) construction
  line L5 (-27.15, 22) -> (-27.15, 43.3) construction
  line L6 (-27.15, 22) -> (-72.85, 22)
  line L7 (-72.85, 22) -> (-72.85, 32)
  line L8 (-72.85, 32) -> (-27.15, 32)
  line L9 (-27.15, 32) -> (-27.15, 22)
  dimension "d111" = 22.85
  dimension "d112" = 21.3
  dimension "d113" = 45.7
  dimension "d114" = 10
  constraint midpoint L2 L4.start
  constraint perpendicular L1 L4
  constraint perpendicular L2 L5
  constraint horizontal L6
  constraint vertical L7
  constraint horizontal L8
  constraint vertical L9
  measures "d111" distance of L4.start L4.end
  measures "d112" distance of L4.end L5.end
  measures "d113" distance of L4.end L6.end
  measures "d114" distance of L6.end L7.end
extrude "Extrude2'''" add sketch "Sketch3 (2)" against normal blind 3 contours L2 L6 L7 L8 L9 bodies 10 in component "Ultrasonic_Sensor_Mount"
sketch "Sketch4 (2)" plane through (-3, 0, 0) normal (-1, 0, 0) x (0, 0, 1) in component "Ultrasonic_Sensor_Mount"
  circle A0 centre (-50, -6.65) radius 1.375
  circle A1 centre (-50, -11.65) radius 1.375
  line L0 (-53, -14) -> (-47, -14)
  line L1 (-47, -14) -> (-47, 22)
  line L2 (-47, 22) -> (-27.15, 22)
  line L3 (-27.15, 22) -> (-27.15, 32)
  line L4 (-27.15, 32) -> (-72.85, 32)
  line L5 (-72.85, 32) -> (-72.85, 22)
  line L6 (-72.85, 22) -> (-53, 22)
  line L7 (-53, 22) -> (-53, -14)
  line L8 (-47, 22) -> (-53, 22)
  constraint coincident L1.end L2.start
  constraint coincident L6.end L7.start
extrude "Extrude3'" add sketch "Sketch4 (2)" along normal blind 5 contours L2 L3 L4 L5 L6 L8 bodies 10 in component "Ultrasonic_Sensor_Mount"
extrude "Extrude4'" add 1 faces at (-2.6667, 32, -42.3833) along direction (0, 1, 0) blind 11.3 on bodies 10 bodies 10 in component "Ultrasonic_Sensor_Mount"
fillet "Fillet1''" radius 5 3 edges at (-1.5, 22, -53) (-3, 22, -50) (-1.5, 22, -47) on bodies 10 in component "Ultrasonic_Sensor_Mount"
sketch "Sketch5 (2)" plane through (-8, 0, 0) normal (-1, 0, 0) x (0, 0, 1) in component "Ultrasonic_Sensor_Mount"
  line L0 (-27.15, 22) -> (-27.15, 43.3)
  line L1 (-27.15, 43.3) -> (-72.85, 43.3)
  line L2 (-72.85, 43.3) -> (-72.85, 22)
  line L3 (-72.85, 22) -> (-58, 22)
  line L4 (-58, 22) -> (-42, 22)
  line L5 (-42, 22) -> (-27.15, 22)
  line L6 (-72.85, 22) -> (-70.35, 22) construction
  line L7 (-70.35, 22) -> (-70.35, 24.5) construction
  line L8 (-70.35, 24.5) -> (-72.85, 24.5) construction
  line L9 (-72.85, 24.5) -> (-72.85, 22) construction
  circle A0 centre (-70.35, 24.5) radius 2
  line L10 (-27.15, 43.3) -> (-29.65, 43.3) construction
  line L11 (-29.65, 43.3) -> (-29.65, 40.8) construction
  line L12 (-29.65, 40.8) -> (-27.15, 40.8) construction
  line L13 (-27.15, 40.8) -> (-27.15, 43.3) construction
  circle A1 centre (-29.65, 40.8) radius 2
  dimension "d122" = 2.5
  dimension "d123" = 2.5
  dimension "d124" = 4
  dimension "d125" = 2.5
  dimension "d126" = 2.5
  dimension "d127" = 4
  constraint horizontal L6
  constraint vertical L7
  constraint horizontal L8
  constraint vertical L9
  constraint coincident L2.end L3.start
  constraint coincident L7.end L8.start
  constraint horizontal L10
  constraint vertical L11
  constraint horizontal L12
  constraint vertical L13
  constraint coincident L0.end L1.start
  constraint coincident L11.end L12.start
  measures "d122" distance of L6.end L7.end
  measures "d123" distance of L7.end L8.end
  measures "d124" diameter of A0
  measures "d125" distance of L0.end L10.end
  measures "d126" distance of L0.end L12.end
  measures "d127" diameter of A1
extrude "Extrude5'" cut sketch "Sketch5 (2)" against normal blind 8 contours A0 | A1 bodies 10 in component "Ultrasonic_Sensor_Mount"
sketch "Sketch6" plane through (-8, 0, 0) normal (-1, 0, 0) x (0, 0, 1) in component "Ultrasonic_Sensor_Mount"
  circle A0 centre (-70.35, 24.5) radius 2
  circle A1 centre (-29.65, 40.8) radius 2
  line L0 (-27.15, 22) -> (-27.15, 43.3)
  line L1 (-27.15, 43.3) -> (-72.85, 43.3)
  line L2 (-72.85, 43.3) -> (-72.85, 22)
  line L3 (-72.85, 22) -> (-58, 22)
  line L4 (-58, 22) -> (-42, 22)
  line L5 (-42, 22) -> (-27.15, 22)
  line L6 (-67, 22) -> (-67, 43.3)
  line L7 (-67, 43.3) -> (-33, 43.3)
  line L8 (-33, 43.3) -> (-33, 22)
  line L9 (-33, 22) -> (-67, 22)
  line L10 (-33, 26) -> (-67, 26)
  constraint coincident L3 L6.start
  constraint coincident L1 L6.end
  constraint perpendicular L1 L6
  constraint coincident L1 L7.end
  constraint coincident L5 L8.end
  constraint perpendicular L5 L8
  constraint coincident L8 L10.start
  constraint coincident L6 L10.end
  constraint perpendicular L6 L10
extrude "Extrude6'" cut sketch "Sketch6" against normal blind 8 contours L1 L6 L7 L8 L10 bodies 10 in component "Ultrasonic_Sensor_Mount"
fillet "Fillet2'" radius 12.5 2 edges at (-4, 26, -67) (-4, 26, -33) on bodies 10 in component "Ultrasonic_Sensor_Mount"
sketch "Sketch17" plane through (0, -26.65, 0) normal (0, -1, 0) x (1, 0, 0) in component "Chassis"
  line L0 (127.5, -73.5) -> (124.5, -73.5)
  line L1 (124.5, -73.5) -> (124.5, -68.5)
  line L2 (124.5, -68.5) -> (127.5, -68.5)
  line L3 (127.5, -68.5) -> (127.5, -73.5)
  line L4 (183.5, -73.5) -> (180.5, -73.5)
  line L5 (180.5, -73.5) -> (180.5, -68.5)
  line L6 (180.5, -68.5) -> (183.5, -68.5)
  line L7 (183.5, -68.5) -> (183.5, -73.5)
  line L8 (127.5, -31.5) -> (124.5, -31.5)
  line L9 (124.5, -31.5) -> (124.5, -26.5)
  line L10 (124.5, -26.5) -> (127.5, -26.5)
  line L11 (127.5, -26.5) -> (127.5, -31.5)
  line L12 (183.5, -31.5) -> (180.5, -31.5)
  line L13 (180.5, -31.5) -> (180.5, -26.5)
  line L14 (180.5, -26.5) -> (183.5, -26.5)
  line L15 (183.5, -26.5) -> (183.5, -31.5)
  arc A0 (157, -3) -> (154, 0) centre (154, -3) ccw
  line L16 (154, 0) -> (3, 0)
  arc A1 (3, 0) -> (0, -3) centre (3, -3) ccw
  line L17 (0, -3) -> (0, -97)
  arc A2 (0, -97) -> (3, -100) centre (3, -97) ccw
  line L18 (3, -100) -> (154, -100)
  arc A3 (154, -100) -> (157, -97) centre (154, -97) ccw
  line L19 (157, -97) -> (157, -94)
  arc A4 (160, -91) -> (157, -94) centre (160, -94) ccw
  line L20 (160, -91) -> (181.27, -91)
  arc A5 (181.27, -91) -> (184.27, -88) centre (181.27, -88) ccw
  line L21 (184.27, -88) -> (184.27, -12)
  arc A6 (184.27, -12) -> (181.27, -9) centre (181.27, -12) ccw
  line L22 (181.27, -9) -> (160, -9)
  arc A7 (157, -6) -> (160, -9) centre (160, -6) ccw
  line L23 (157, -6) -> (157, -3)
  line L24 (36.83, -3.81) -> (36.83, -13.97)
  line L25 (36.83, -13.97) -> (19.05, -13.97)
  line L26 (19.05, -13.97) -> (19.05, -3.81)
  line L27 (19.05, -3.81) -> (36.83, -3.81)
  line L28 (36.83, -96.52) -> (19.05, -96.52)
  line L29 (19.05, -96.52) -> (19.05, -86.36)
  line L30 (19.05, -86.36) -> (36.83, -86.36)
  line L31 (36.83, -86.36) -> (36.83, -96.52)
  line L32 (114.3, -3.81) -> (130.81, -3.81)
  line L33 (130.81, -3.81) -> (130.81, -13.97)
  line L34 (130.81, -13.97) -> (114.3, -13.97)
  line L35 (114.3, -13.97) -> (114.3, -3.81)
  line L36 (114.3, -96.52) -> (114.3, -86.36)
  line L37 (114.3, -86.36) -> (130.81, -86.36)
  line L38 (130.81, -86.36) -> (130.81, -96.52)
  line L39 (130.81, -96.52) -> (114.3, -96.52)
  line L40 (7, -7) -> (16, -7)
  line L41 (16, -7) -> (16, -27.03)
  line L42 (16, -27.03) -> (7, -27.03)
  line L43 (7, -27.03) -> (7, -7)
  line L44 (7, -72.97) -> (16, -72.97)
  line L45 (16, -72.97) -> (16, -93)
  line L46 (16, -93) -> (7, -93)
  line L47 (7, -93) -> (7, -72.97)
  line L48 (16, -82.985) -> (7, -82.985) construction
  line L49 (11.5, -82.985) -> (11.5, -70.07) construction
  line L50 (11.5, -82.985) -> (11.5, -95.9) construction
  circle A8 centre (11.5, -70.07) radius 1
  circle A9 centre (11.5, -95.9) radius 1
  line L51 (16, -17.015) -> (7, -17.015) construction
  line L52 (11.5, -17.015) -> (11.5, -4.1) construction
  line L53 (11.5, -17.015) -> (11.5, -29.93) construction
  circle A10 centre (11.5, -4.1) radius 1
  circle A11 centre (11.5, -29.93) radius 1
  line L54 (112.5, -27.97) -> (92.5, -27.97)
  line L55 (92.5, -27.97) -> (92.5, -18.97)
  line L56 (92.5, -18.97) -> (112.5, -18.97)
  line L57 (112.5, -18.97) -> (112.5, -27.97)
  line L58 (112.5, -27.97) -> (92.5, -18.97) construction
  line L59 (92.5, -27.97) -> (112.5, -18.97) construction
  line L60 (112.5, -81.36) -> (92.5, -81.36)
  line L61 (92.5, -81.36) -> (92.5, -72.36)
  line L62 (92.5, -72.36) -> (112.5, -72.36)
  line L63 (112.5, -72.36) -> (112.5, -81.36)
  line L64 (112.5, -81.36) -> (92.5, -72.36) construction
  line L65 (92.5, -81.36) -> (112.5, -72.36) construction
  line L66 (102.5, -23.47) -> (115.415, -23.47) construction
  line L67 (102.5, -23.47) -> (89.585, -23.47) construction
  line L68 (102.5, -76.86) -> (115.415, -76.86) construction
  line L69 (102.5, -76.86) -> (89.585, -76.86) construction
  circle A12 centre (89.585, -23.47) radius 1
  circle A13 centre (115.415, -23.47) radius 1
  circle A14 centre (89.585, -76.86) radius 1
  circle A15 centre (115.415, -76.86) radius 1
  point P0 (102.5, -23.47)
  point P1 (102.5, -76.86)
  dimension "d133" = 20.03
  dimension "d134" = 9
  dimension "d135" = 20.03
  dimension "d136" = 9
  dimension "d137" = 7
  dimension "d138" = 7
  dimension "d139" = 7
  dimension "d140" = 7
  dimension "d141" = 12.915
  dimension "d142" = 12.915
  dimension "d143" = 2
  dimension "d144" = 2
  dimension "d145" = 12.915
  dimension "d146" = 12.915
  dimension "d147" = 2
  dimension "d148" = 2
  dimension "d149" = 20
  dimension "d150" = 9
  dimension "d151" = 20
  dimension "d152" = 9
  dimension "d153" = 12
  dimension "d154" = 12
  dimension "d155" = 5
  dimension "d156" = 5
  dimension "d157" = 12.915
  dimension "d158" = 12.915
  dimension "d159" = 12.915
  dimension "d160" = 12.915
  dimension "d161" = 2
  dimension "d162" = 2
  dimension "d163" = 2
  dimension "d164" = 2
  constraint horizontal L40
  constraint vertical L41
  constraint horizontal L42
  constraint vertical L43
  constraint horizontal L44
  constraint vertical L45
  constraint horizontal L46
  constraint vertical L47
  constraint midpoint L45 L48.start
  constraint midpoint L47 L48.end
  constraint midpoint L48 L49.start
  constraint perpendicular L44 L49
  constraint perpendicular L48 L50
  constraint coincident L49.end A8.centre
  constraint coincident L50.end A9.centre
  constraint midpoint L41 L51.start
  constraint midpoint L43 L51.end
  constraint midpoint L51 L52.start
  constraint perpendicular L40 L52
  constraint perpendicular L42 L53
  constraint coincident L52.end A10.centre
  constraint coincident L53.end A11.centre
  constraint horizontal L54
  constraint perpendicular L54 L55
  constraint parallel L54 L56
  constraint parallel L55 L57
  constraint coincident L58 P0
  constraint coincident L59 P0
  constraint horizontal L60
  constraint perpendicular L60 L61
  constraint parallel L60 L62
  constraint parallel L61 L63
  constraint coincident L64 P1
  constraint coincident L65 P1
  constraint coincident P0 L66.start
  constraint horizontal L66
  constraint parallel L66 L67
  constraint coincident P1 L68.start
  constraint perpendicular L63 L68
  constraint parallel L68 L69
  constraint coincident L67.end A12.centre
  constraint coincident L66.end A13.centre
  constraint coincident L69.end A14.centre
  constraint coincident L68.end A15.centre
  measures "d133" distance of L40.start L42.end
  measures "d134" distance of L40.start L40.end
  measures "d135" distance of L44.start L46.end
  measures "d136" distance of L44.start L44.end
  measures "d137" distance of L17 L43
  measures "d138" distance of L16 L40
  measures "d139" distance of L18 L46
  measures "d140" distance of L17 L47
  measures "d141" distance of L49.start L49.end
  measures "d142" distance of L49.start L50.end
  measures "d143" diameter of A8
  measures "d144" diameter of A9
  measures "d145" distance of L52.start L52.end
  measures "d146" distance of L52.start L53.end
  measures "d147" diameter of A10
  measures "d148" diameter of A11
  measures "d149" distance of L55.end L56.end
  measures "d150" distance of L54.end L55.end
  measures "d151" distance of L61.end L62.end
  measures "d152" distance of L60.end L61.end
  measures "d153" distance of L9 L57
  measures "d154" distance of L1 L63
  measures "d155" distance of L37 L60
  measures "d156" distance of L34 L56
  measures "d157" distance of P0 L66.end
  measures "d158" distance of P0 L67.end
  measures "d159" distance of P1 L68.end
  measures "d160" distance of P1 L69.end
  measures "d161" diameter of A12
  measures "d162" diameter of A13
  measures "d163" diameter of A14
  measures "d164" diameter of A15
extrude "Extrude16" cut sketch "Sketch17" against normal blind 3 contours L40 L41 L42 L43 | L44 L45 L46 L47 | A8 | A9 | A10 | A11 | L54 L55 L56 L57 | L60 L61 L62 L63 | A12 | A13 | A14 | A15 bodies 4 in component "Chassis"